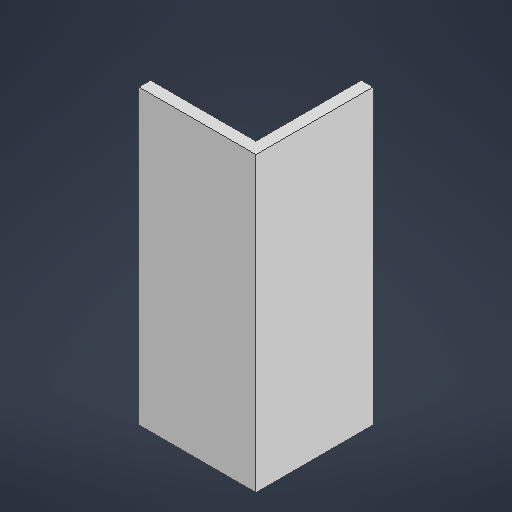
# Autodesk Inventor part: Flower Box Stack Half
Saved by Autodesk Inventor 2025 (Build 290162000, 162)
## iProperties
Created: 2024-07-01
Part Number: Flower Box Stack Half
Material: Generic
Document SubType Name: Modeling
Designer: AlexM
Density: 1 g/cm^3
Appearance: Default
Author: AlexM
Autodesk Inventor part; units mm, degrees
ref_plane "YZ Plane" through (0, 0, 0) normal (1, 0, 0) x (0, 1, 0)
ref_plane "XZ Plane" through (0, 0, 0) normal (0, 1, 0) x (-1, 0, 0)
ref_plane "XY Plane" through (0, 0, 0) normal (0, 0, 1) x (1, 0, 0)
sketch "Sketch1" plane through (0, 0, 0) normal (0, 1, 0) x (-1, 0, 0)
  line L0 (0, 0) -> (5.08, 0)
  line L1 (5.08, 0) -> (5.08, 50.8)
  line L2 (5.08, 50.8) -> (0, 50.8)
  line L3 (0, 50.8) -> (0, 0)
  line L4 (5.08, 50.8) -> (50.8, 50.8)
  line L5 (50.8, 50.8) -> (50.8, 45.72)
  line L6 (50.8, 45.72) -> (5.08, 45.72)
  line L7 (5.08, 45.72) -> (5.08, 50.8)
  point P0 (5.08, 45.72)
  dimension "d5" = 50.8
  dimension "d6" = 5.08
  dimension "d7" = 5.08
  dimension "d8" = 50.8
  constraints: 16 end point, 4 parallel, 2 horizontal, 2 perpendicular
  measures "d5" distance of L0.end L1.end
  measures "d6" distance of L1.end L2.end
  measures "d7" distance of L4.end L5.end
  measures "d8" distance between parallel lines of L3 L5
extrude "Extrusion1" add sketch "Sketch1" along normal blind 127
body "Solid1"
